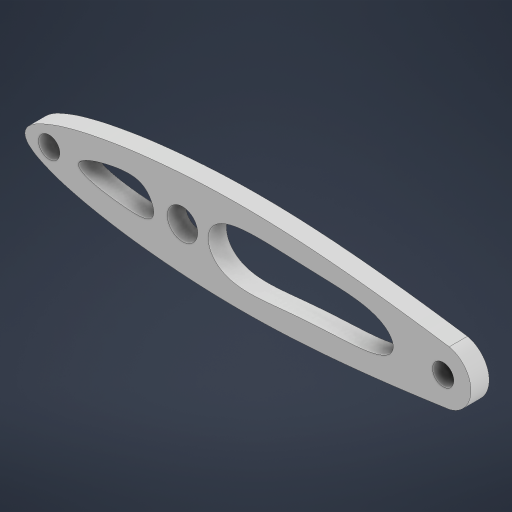
# Autodesk Inventor part: Tżebro z lotkąt
Saved by Autodesk Inventor 2023.2 (Build 272271000, 271)
## iProperties
Created: 2022-12-28
Part Number: Tżebro z lotkąt
Material: Generic
Document SubType Name: Modeling
Designer: Maciej
Density: 1 g/cm^3
Appearance: Default
Author: Maciej
Autodesk Inventor part; units mm, degrees
ref_plane "YZ Plane" through (0, 0, 0) normal (1, 0, 0) x (0, 1, 0)
ref_plane "XZ Plane" through (0, 0, 0) normal (0, 1, 0) x (-1, 0, 0)
ref_plane "XY Plane" through (0, 0, 0) normal (0, 0, 1) x (1, 0, 0)
sketch "Sketch1" plane through (0, 0, 0) normal (0, 0, 1) x (1, 0, 0)
  spline S0 degree 4 poles (100, 0.032) (96.875, 0.4949) (92.5, 1.1413) (86.8751, 1.9754) (80.0002, 2.991) (75.0008, 3.7295) (70.0033, 4.4751) (65.0053, 5.1842) (60.0066, 5.8364) (55.0071, 6.4061) (50.0063, 6.8809) (45.0061, 7.2433) (40.0008, 7.4683) (35.0047, 7.533) (29.9791, 7.4197) (25.0319, 7.1346) (19.9582, 6.6428) (15.6359, 6.1039) (10.2184, 5.101) (7.8303, 4.4733) (5.3127, 3.8052) (2.8544, 2.7785) (1.5003, 2.0987) (0.6956, 1.3847) (0.5171, 1.2937) (-0.3402, 0) (0.5171, -1.2937) (0.6956, -1.3847) (1.5003, -2.0987) (2.8544, -2.7785) (5.3127, -3.8052) (7.8303, -4.4733) (10.2184, -5.101) (15.6359, -6.1039) (19.9582, -6.6428) (25.0319, -7.1346) (29.9791, -7.4197) (35.0047, -7.533) (40.0008, -7.4683) (45.0061, -7.2433) (50.0063, -6.8809) (55.0071, -6.4061) (60.0066, -5.8364) (65.0053, -5.1842) (70.0033, -4.4751) (75.0008, -3.7295) (80.0002, -2.991) (86.8751, -1.9754) (92.5, -1.1413) (96.875, -0.4949) (100, -0.032) knots 0 0 0 0 0 0.057355 0.080296 0.103238 0.126177 0.149108 0.172027 0.194928 0.217807 0.240666 0.263507 0.286336 0.309162 0.331999 0.354861 0.377772 0.399068 0.418771 0.436942 0.45243 0.465861 0.476678 0.486208 0.495579 0.504421 0.513792 0.523322 0.534139 0.54757 0.563058 0.581229 0.600932 0.622228 0.645139 0.668001 0.690838 0.713664 0.736493 0.759334 0.782193 0.805072 0.827973 0.850892 0.873823 0.896762 0.919704 0.942645 1 1 1 1 1
  circle A0 centre (26, 0) radius 2.5
  circle A1 centre (4, 0) radius 1.75
  circle A2 centre (69, 0) radius 1.75
  spline S1 degree 5 poles (8.9035, 0.2296) (9.2434, 0.8899) (11.3643, 2.0291) (18.2315, 3.5428) (20.2721, 2.9595) (23.0162, -3.0821) (16.5301, -2.3219) (12.7289, -2.0151) (9.2115, -1.112) (8.6356, -0.2907) (8.9035, 0.2296) knots 0 0 0 0 0 0 0.227523 0.364622 0.543771 0.698813 0.820709 1 1 1 1 1 1
  spline S2 degree 5 poles (31.2707, 2.5) (32.7339, 3.9218) (37.2285, 5.1212) (48.2817, 2.605) (61.2094, 6.6741) (64.3828, -5.6022) (45.0929, -1.179) (33.1446, -7.1128) (29.4849, -1.5962) (30.0097, 1.2748) (31.2707, 2.5) knots 0 0 0 0 0 0 0.215917 0.355077 0.532597 0.692902 0.813935 1 1 1 1 1 1
  line L0 (100, -0.032) -> (100.1, 0)
  line L1 (100.1, 0) -> (100, 0.032)
  circle A3 centre (69, 0) radius 4.5785
  line L2 (75, 3.731) -> (79.9461, 2.999)
  line L3 (79.9461, 2.999) -> (79.6826, 1.2184)
  line L4 (79.6826, 1.2184) -> (74.7365, 1.9504)
  line L5 (74.7365, 1.9504) -> (75, 3.731)
  line L6 (80, -2.991) -> (84.9463, -2.2599)
  line L7 (84.9463, -2.2599) -> (84.6831, -0.4793)
  line L8 (84.6831, -0.4793) -> (79.7368, -1.2103)
  line L9 (79.7368, -1.2103) -> (80, -2.991)
  point P0 (0, 0)
  point P1 (95, 0.772)
  point P2 (90, 1.512)
  point P3 (85, 2.252)
  point P4 (80, 2.991)
  point P5 (70, 4.468)
  point P6 (65, 5.173)
  point P7 (60, 5.82)
  point P8 (55, 6.387)
  point P9 (50, 6.858)
  point P10 (45, 7.215)
  point P11 (40, 7.435)
  point P12 (35, 7.496)
  point P13 (30, 7.384)
  point P14 (25, 7.091)
  point P15 (20, 6.619)
  point P16 (15, 5.942)
  point P17 (10, 4.997)
  point P18 (7.5, 4.382)
  point P19 (5, 3.618)
  point P20 (2.5, 2.579)
  point P21 (1.25, 1.844)
  point P22 (0.75, 1.448)
  point P23 (0.5, 1.203)
  point P24 (0, 0)
  point P25 (0.5, -1.203)
  point P26 (0.75, -1.448)
  point P27 (1.25, -1.844)
  point P28 (2.5, -2.579)
  point P29 (5, -3.618)
  point P30 (7.5, -4.382)
  point P31 (10, -4.997)
  point P32 (15, -5.942)
  point P33 (20, -6.619)
  point P34 (25, -7.091)
  point P35 (30, -7.384)
  point P36 (35, -7.496)
  point P37 (40, -7.435)
  point P38 (45, -7.215)
  point P39 (50, -6.858)
  point P40 (55, -6.387)
  point P41 (60, -5.82)
  point P42 (65, -5.173)
  point P43 (70, -4.468)
  point P44 (75, -3.731)
  point P45 (80, -2.991)
  point P46 (85, -2.252)
  point P47 (90, -1.512)
  point P48 (95, -0.772)
  point P49 (20.5674, 1.203)
  point P50 (21.0369, -1.512)
  point P51 (16.8986, -2.3616)
  point P52 (10, -1.1013)
  point P53 (59.6934, 1.7909)
  point P54 (60.4025, -1.203)
  point P55 (44.4534, -3.7857)
  point P56 (31.0165, -2.1426)
  point P57 (70, -4.468)
  dimension "d0" = 5
  dimension "d1" = 3.5
  dimension "d2" = 3.5
  dimension "d3" = 26
  dimension "d4" = 22
  dimension "d5" = 43
  dimension "d6" = 0.1
  dimension "d9" = 5
  dimension "d10" = 1.8
  dimension "d11" = 5
  dimension "d12" = 1.8
  constraints: 20 end point, 4 parallel, 3 centre point, 3 horizontal alignment, 2 perpendicular, 1 coincident, 121 other
  measures "d0" diameter of A0
  measures "d1" diameter of A1
  measures "d2" diameter of A2
  measures "d3" distance of A0.centre point (0, 0)
  measures "d4" distance of A0.centre A1.centre
  measures "d5" distance of A2.centre A0.centre
  measures "d6" horizontal distance of L1.end L0.end
  measures "d9" distance of L2.start L2.end
  measures "d10" distance of L2.end L3.end
  measures "d11" distance of L6.start L6.end
  measures "d12" distance of L7.end L6.end
extrude "Extrusion1" add sketch "Sketch1" along normal blind 3 contours A3 S0 | A3 S0 picked at (65.4059, -0.3539) picked at (48.6012, -4.5374)
body "Solid1"
